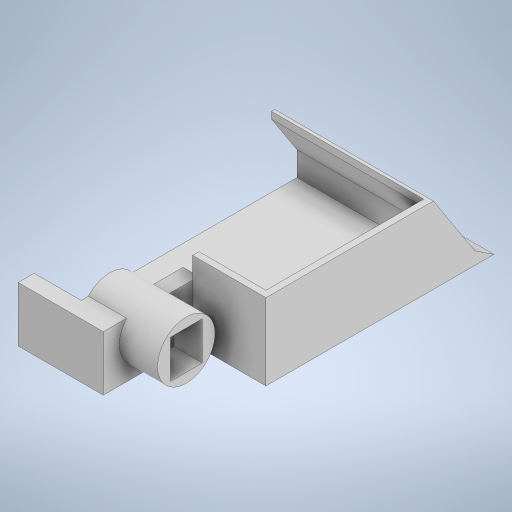
# Autodesk Inventor part: Tělo
Saved by Autodesk Inventor 2024 (Build 280153000, 153)
## iProperties
Created: 2023-04-15
Part Number: Tělo
Material: Všeobecné
Document SubType Name: Modeling
Designer: 42060
Density: 1 g/cm^3
Appearance: Výchozí
Author: 42060
Autodesk Inventor part; units mm, degrees
ref_plane "YZ Plane" through (0, 0, 0) normal (1, 0, 0) x (0, 1, 0)
ref_plane "XZ Plane" through (0, 0, 0) normal (0, 1, 0) x (-1, 0, 0)
ref_plane "XY Plane" through (0, 0, 0) normal (0, 0, 1) x (1, 0, 0)
sketch "Základ" plane through (0, 0, 0) normal (0, 0, 1) x (1, 0, 0)
  line L0 (0, 0) -> (49.75, 0)
  line L1 (49.75, 0) -> (49.75, -71.5)
  line L2 (49.75, -71.5) -> (26.75, -71.5)
  line L3 (26.75, -99.5) -> (0, -99.5)
  line L4 (0, -99.5) -> (0, 0)
  line L5 (0, -20) -> (47.75, -20)
  line L6 (47.75, -20) -> (47.75, -69.5)
  line L7 (47.75, -69.5) -> (21.75, -69.5)
  line L8 (21.75, -69.5) -> (21.75, -94.5)
  line L9 (21.75, -94.5) -> (0, -94.5)
  line L10 (26.75, -71.5) -> (26.75, -80.5)
  line L11 (26.75, -80.5) -> (26.75, -90.5)
  line L12 (26.75, -90.5) -> (26.75, -99.5)
  line L13 (26.75, -90.5) -> (21.75, -90.5)
  line L14 (26.75, -80.5) -> (21.75, -80.5)
  line L15 (26.75, -71.5) -> (26.75, -69.5)
  dimension "d0" = 49.75
  dimension "d1" = 99.5
  dimension "d3" = 2
  dimension "d5" = 28
  dimension "d14" = 10
  dimension "d15" = 5
  dimension "d16" = 5
  dimension "d17" = 23
  dimension "d18" = 2
  dimension "d19" = 20
  constraints: 32 end point, 8 perpendicular, 6 point on line, 3 horizontal, 2 collinear, 1 parallel, 1 vertical
  measures "d0" distance of L0.start L0.end
  measures "d1" distance between parallel lines of L3 L0
  measures "d3" distance between parallel lines of L1 L6
  measures "d5" distance of L2.end L3.start
  measures "d14" distance of L10.end L11.end
  measures "d15" distance between parallel lines of L8 L10
  measures "d16" distance between parallel lines of L9 L3
  measures "d17" distance between parallel lines of L1 L12
  measures "d18" distance between parallel lines of L2 L7
  measures "d19" distance between parallel lines of L0 L5
extrude "Podlaha" add sketch "Základ" along normal blind 2 contours L5 L6 L7 L8 L9 L4
extrude "Stěny" add sketch "Základ" along normal blind 24 contours L0 L1 L2 L15 L7 L6 L5 L4
extrude "Zadní stěny" add sketch "Základ" along normal blind 17.25 contours L9 L8 L13 L12 L3 L4 | L10 L14 L8 L7 L15
extrude "Stěna pod motorem" add sketch "Základ" along normal blind 5.25 contours L11 L13 L8 L14
sketch "Náčrt2" plane through (49.75, -71.5, 0) normal (1, 0, 0) x (0, 0, -1)
  line L0 (-2, 51.5) -> (-24, 51.5) projected
  line L1 (-2, 51.5) -> (-24, 51.5) projected
  line L2 (-24, 0) -> (-24, 71.5) projected
  line L3 (0, 71.5) -> (-24, 71.5) projected
  line L4 (0, 71.5) -> (0, 0) projected
  line L5 (-24, 52.5) -> (-4, 65.5)
  line L6 (-4, 65.5) -> (0, 71.5)
  dimension "d28" = 1
  dimension "d29" = 6
  dimension "d30" = 20
  constraints: 4 end point, 1 point on line
  measures "d28" distance from line of L5.start L0
  measures "d29" vertical distance of L3.start L5.end
  measures "d30" horizontal distance of L5.end L5.start
extrude "Rampa" cut sketch "Náčrt2" against normal through all
sketch "Náčrt3" plane through (0, -20, 2) normal (-1, 0, 0) x (0, 0, 1)
  line L0 (0, 0) -> (22, 0) projected
  line L1 (0, 0) -> (22, 0) projected
  line L2 (19.8687, 0) -> (7.5, 8.0396)
  line L3 (7.5, 8.0396) -> (0, 8.0396)
  line L4 (0, 8.0396) -> (0, 0)
  line L5 (22, 1) -> (2, 14) projected
  point P0 (-2, 20)
  point P1 (19.8687, 0)
  dimension "d34" = 7.5
  dimension "d37" = 2
  constraints: 6 end point, 1 horizontal, 1 parallel, 1 perpendicular, 1 point on line
  measures "d34" distance of L2.end L3.end
  measures "d37" distance between parallel lines of L2 L5
extrude "Vysunutí6" cut sketch "Náčrt3" against normal up to surface (47.75 mm away)
sketch "Náčrt4" plane through (21.75, -94.5, 2) normal (-1, 0, 0) x (0, 0, 1)
  line L0 (3.25, 14) -> (15.25, 14) projected
  line L1 (3.25, 14) -> (3.25, 4) projected
  line L2 (3.25, 4) -> (15.25, 4) projected
  line L3 (5.9334, 14) -> (12.5666, 14)
  line L4 (12.5666, 4) -> (5.9334, 4)
  line L5 (3.25, 4) -> (15.25, 4) projected
  arc A0 (12.5666, 4) -> (12.5666, 14) centre (9.25, 9) ccw
  arc A1 (5.9334, 14) -> (5.9334, 4) centre (9.25, 9) ccw
  line L6 (15.25, 14) -> (15.25, 4) construction
  circle A2 centre (9.25, 9) radius 9
  line L7 (9.25, 18) -> (0, 18)
  line L8 (0, 0) -> (0, 82.5396) projected
  line L9 (15.25, 2.2918) -> (15.25, 0)
  line L10 (0, 0) -> (15.25, 0) projected
  point P0 (-2, 94.5)
  point P1 (15.25, 9)
  point P2 (15.25, 9)
  point P3 (3.25, 9)
  point P4 (3.25, 9)
  point P5 (5.9334, 4)
  point P6 (9.25, 0)
  dimension "d38" = 6
  dimension "d39" = 6
  dimension "d41" = 3
  constraints: 10 end point, 8 point on circle, 5 point on line, 3 centre point, 3 coincident, 3 tangent, 2 midpoint, 2 vertical, 1 horizontal
  measures "d38" radius of A0
  measures "d39" radius of A1
  measures "d41" radial gap between concentric circles of A2 A0
extrude "Vysunutí7" add sketch "Náčrt4" against normal blind 8 contours L0 A1 L1 | A1 L2 L1 | A2
sketch "Náčrt5" plane through (29.75, -85.5, 11.25) normal (1, 0, 0) x (0, 0, -1)
  line L0 (-6, 5) -> (6, 5)
  line L1 (6, 5) -> (6, -5)
  line L2 (6, -5) -> (-6, -5)
  line L3 (-6, -5) -> (-6, 5)
  line L4 (-6, 5) -> (6, -5) construction
  line L5 (6, 5) -> (-6, -5) construction
  arc A0 (3.3166, -5) -> (3.3166, 5) centre (0, 0) ccw projected
  arc A1 (-3.3166, 5) -> (-3.3166, -5) centre (0, 0) ccw projected
  line L6 (3.3166, -5) -> (-3.3166, -5) projected
  line L7 (-3.3166, 5) -> (3.3166, 5) projected
  circle A2 centre (0, 0) radius 9 projected
  point P0 (11.25, 85.5)
  point P1 (0, 0)
  constraints: 12 end point, 2 collinear, 2 midpoint, 2 parallel, 2 tangent, 1 horizontal, 1 perpendicular
extrude "Vysunutí8" add sketch "Náčrt5" along normal blind 9
extrude "Vysunutí9" add sketch "Náčrt4" along normal blind 7 contours L0 A1 L1 | A1 L2 L1 | A2 | A2 L10 L8 L7 | L9 L10 A2
